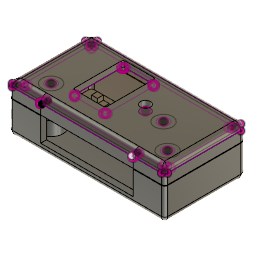
Diag_CP v4 (Autodesk Fusion 360 design; units mm, degrees)
Autodesk Fusion 360 part; units mm, degrees
sketch "Skizze1" plane through (0, 0, 0) normal (0, 0, 1) x (1, 0, 0)
  line L0 (14.5161, 23.538) -> (14.5161, 23.6029)
  line L1 (14.5161, 23.6029) -> (14.581, 23.6029)
  arc A0 (15.5262, 23.0188) -> (15.3315, 23.2135) centre (15.3315, 23.0188) ccw
  line L2 (16.0356, 22.6293) -> (16.0356, 23.0188)
  arc A1 (16.0356, 22.6293) -> (16.2303, 22.4346) centre (16.2303, 22.6293) ccw
  line L3 (16.2303, 23.2135) -> (16.5549, 23.2135)
  line L4 (13.7104, 22.4346) -> (13.3858, 22.4346)
  arc A2 (0, 1) -> (1, 0) centre (1, 1) ccw
  line L5 (14.0349, 23.2784) -> (14.0349, 22.7591)
  arc A3 (14.035, 23.2784) -> (13.7104, 23.603) centre (13.7104, 23.2784) ccw
  line L6 (15.3315, 23.2135) -> (15.0718, 23.2135)
  arc A4 (16.2303, 23.2135) -> (16.0356, 23.0188) centre (16.2303, 23.0188) ccw
  line L7 (16.3602, 22.0451) -> (16.1005, 22.0451)
  arc A5 (1, 25) -> (0, 24) centre (1, 24) ccw
  line L8 (15.2341, 22.4346) -> (15.5262, 22.4346)
  line L9 (30, 24) -> (30, 1)
  arc A6 (15.2341, 22.8889) -> (15.2341, 22.4345) centre (15.2341, 22.6617) ccw
  arc A7 (16.3602, 22.0451) -> (16.5549, 22.2398) centre (16.3602, 22.2398) ccw
  line L10 (16.5549, 22.4346) -> (16.2303, 22.4346)
  line L11 (14.5486, 22.4346) -> (14.5486, 23.2135)
  arc A8 (30, 24) -> (29, 25) centre (29, 24) ccw
  line L12 (14.581, 23.6029) -> (14.581, 23.538)
  line L13 (16.5549, 23.2135) -> (16.5549, 22.2398)
  line L14 (29, 0) -> (1, 0)
  line L15 (13.3858, 23.6029) -> (13.7104, 23.6029)
  line L16 (17.6911, 22.4346) -> (18.0806, 22.4346)
  line L17 (13.3858, 22.4346) -> (13.3858, 23.6029)
  line L18 (14.581, 23.538) -> (14.5161, 23.538)
  arc A9 (29, 0) -> (30, 1) centre (29, 1) ccw
  line L19 (0, 1) -> (0, 24)
  line L20 (15.5262, 22.8889) -> (15.2341, 22.8889)
  arc A10 (13.7104, 22.4345) -> (14.035, 22.7591) centre (13.7104, 22.7591) ccw
  line L21 (15.5262, 22.4346) -> (15.5262, 23.0188)
  arc A11 (18.3402, 22.824) -> (18.0806, 23.0836) centre (18.0806, 22.824) ccw
  arc A12 (22.8148, 23.0837) -> (22.9122, 23.3109) centre (22.5984, 23.3109) ccw
  arc A13 (18.834, 22.7591) -> (19.4832, 22.7591) centre (19.1586, 22.7591) ccw
  arc A14 (23.406, 23.0188) -> (23.5034, 22.5969) centre (24.3689, 23.0188) ccw
  line L22 (19.9771, 23.0837) -> (20.3665, 23.0837)
  line L23 (22.2631, 22.4346) -> (22.9122, 22.4346)
  arc A15 (19.4832, 22.7591) -> (18.834, 22.7591) centre (19.1586, 22.7591) ccw
  arc A16 (23.5034, 22.5968) -> (23.7306, 22.4345) centre (23.7306, 22.6747) ccw
  line L24 (1, 25) -> (29, 25)
  arc A17 (21.7692, 23.3109) -> (21.4771, 23.603) centre (21.4771, 23.3109) ccw
  arc A18 (21.4771, 23.603) -> (21.1201, 23.3433) centre (21.4771, 23.2277) ccw
  arc A19 (20.6261, 22.824) -> (20.3665, 23.0836) centre (20.3665, 22.824) ccw
  arc A20 (15.716, 20.6883) -> (15.7809, 21.0129) centre (15.7184, 20.8566) ccw
  line L25 (13.3858, 20.9479) -> (13.3858, 21.5971)
  arc A21 (19.4182, 23.3433) -> (18.899, 23.3433) centre (19.1586, 23.3433) ccw
  line L26 (22.8148, 23.0837) -> (22.2631, 22.4346)
  line L27 (18.3402, 22.6942) -> (18.3402, 22.824)
  line L28 (17.6911, 23.0837) -> (17.6911, 23.6029)
  arc A22 (13.6454, 21.8567) -> (13.3858, 21.5971) centre (13.6454, 21.5971) ccw
  arc A23 (14.5516, 21.1427) -> (14.5516, 20.6883) centre (14.5516, 20.9155) ccw
  arc A24 (17.3403, 20.883) -> (17.535, 20.6883) centre (17.535, 20.883) ccw
  line L29 (17.3402, 20.883) -> (17.3402, 21.2076)
  arc A25 (22.9122, 23.3109) -> (22.6201, 23.603) centre (22.6201, 23.3109) ccw
  line L30 (18.0806, 23.0837) -> (17.6911, 23.0837)
  arc A26 (18.899, 23.3433) -> (19.4182, 23.3433) centre (19.1586, 23.3433) ccw
  line L31 (17.8595, 20.6883) -> (17.535, 20.6883)
  arc A27 (17.8595, 21.2076) -> (17.3403, 21.2076) centre (17.5999, 21.2076) ccw
  arc A28 (23.9578, 23.4407) -> (23.7306, 23.603) centre (23.7306, 23.3628) ccw
  arc A29 (20.4964, 23.603) -> (19.9771, 23.0837) centre (20.4964, 23.0837) ccw
  line L32 (14.5516, 20.6883) -> (14.8437, 20.6883)
  line L33 (21.1201, 22.4346) -> (21.7692, 22.4346)
  line L34 (21.6718, 23.0837) -> (21.1201, 22.4346)
  line L35 (20.6262, 22.824) -> (20.6262, 22.7591)
  line L36 (13.6454, 21.8567) -> (13.9051, 21.8567)
  arc A30 (23.5035, 23.4407) -> (23.4061, 23.0188) centre (24.3689, 23.0188) ccw
  line L37 (17.6911, 23.6029) -> (18.3402, 23.6029)
  line L38 (15.7809, 21.0129) -> (15.4564, 21.1427)
  line L39 (14.8437, 20.6883) -> (14.8437, 21.2725)
  arc A31 (19.977, 22.7591) -> (20.6262, 22.7591) centre (20.3016, 22.7591) ccw
  line L40 (19.9771, 22.7591) -> (19.9771, 23.0837)
  arc A32 (22.6201, 23.603) -> (22.2631, 23.3433) centre (22.6201, 23.2277) ccw
  arc A33 (24.0552, 23.0188) -> (23.9578, 23.4407) centre (23.0923, 23.0188) ccw
  arc A34 (18.0806, 22.4346) -> (18.3402, 22.6942) centre (18.0806, 22.6942) ccw
  arc A35 (23.7306, 23.603) -> (23.5034, 23.4407) centre (23.7306, 23.3628) ccw
  arc A36 (21.6718, 23.0837) -> (21.7692, 23.3109) centre (21.4554, 23.3109) ccw
  arc A37 (19.7787, 20.883) -> (19.9734, 20.6883) centre (19.9734, 20.883) ccw
  line L41 (13.3858, 19.1008) -> (13.3858, 20.2692)
  line L42 (18.958, 21.4672) -> (19.3475, 21.4672)
  line L43 (16.3756, 19.1008) -> (16.3756, 19.1657)
  line L44 (13.7104, 19.6201) -> (13.3858, 19.6201)
  line L45 (20.2979, 21.2076) -> (20.2979, 21.0778)
  line L46 (15.7223, 19.1008) -> (15.9819, 19.8797)
  arc A38 (13.7104, 19.62) -> (13.7104, 20.2692) centre (13.7104, 19.9446) ccw
  line L47 (18.5587, 20.6883) -> (18.6236, 20.6883)
  arc A39 (18.364, 20.883) -> (18.5587, 20.6883) centre (18.5587, 20.883) ccw
  line L48 (14.5101, 19.2955) -> (14.5101, 19.6201)
  line L49 (15.0294, 19.6201) -> (15.0294, 19.4903)
  line L50 (15.0294, 19.1008) -> (14.7049, 19.1008)
  arc A40 (16.7066, 20.6883) -> (16.7715, 21.0129) centre (16.709, 20.8566) ccw
  line L51 (19.2826, 20.6883) -> (19.3475, 20.6883)
  arc A41 (18.045, 20.1069) -> (17.8178, 20.2692) centre (17.8178, 20.029) ccw
  arc A42 (20.2979, 21.2076) -> (19.7787, 21.2076) centre (20.0383, 21.2076) ccw
  arc A43 (23.7306, 22.4345) -> (23.9578, 22.5968) centre (23.7306, 22.6747) ccw
  arc A44 (16.804, 21.4023) -> (16.5119, 21.4672) centre (16.5014, 20.7302) ccw
  line L52 (17.8595, 21.2076) -> (17.8595, 21.0778)
  arc A45 (16.5119, 21.4672) -> (16.447, 21.1426) centre (16.5095, 21.2989) ccw
  line L53 (20.2979, 21.0778) -> (19.7786, 21.0778)
  line L54 (16.4405, 19.1657) -> (16.4405, 19.1008)
  arc A46 (19.0879, 20.883) -> (19.2826, 20.6883) centre (19.2826, 20.883) ccw
  arc A47 (14.5102, 19.2955) -> (14.7049, 19.1008) centre (14.7049, 19.2955) ccw
  line L55 (16.3756, 19.1657) -> (16.4405, 19.1657)
  line L56 (13.9051, 20.6883) -> (13.6454, 20.6883)
  arc A48 (15.3591, 20.7532) -> (15.7161, 20.6883) centre (15.7318, 21.789) ccw
  line L57 (18.2341, 21.4672) -> (18.6236, 21.4672)
  line L58 (14.0349, 19.1008) -> (13.7753, 19.6201)
  line L59 (14.649, 21.4672) -> (14.3894, 21.4672)
  arc A49 (15.8134, 21.4023) -> (15.5213, 21.4672) centre (15.5108, 20.7302) ccw
  arc A50 (14.8437, 21.2725) -> (14.649, 21.4672) centre (14.649, 21.2725) ccw
  arc A51 (16.3497, 20.7532) -> (16.7067, 20.6883) centre (16.7224, 21.789) ccw
  arc A52 (13.3858, 20.9479) -> (13.6454, 20.6883) centre (13.6454, 20.9479) ccw
  line L60 (18.3639, 21.8567) -> (18.3639, 20.883)
  line L61 (17.8595, 21.0778) -> (17.3402, 21.0778)
  arc A53 (23.9578, 22.5969) -> (24.0552, 23.0188) centre (23.0923, 23.0188) ccw
  arc A54 (15.5213, 21.4672) -> (15.4564, 21.1426) centre (15.5189, 21.2989) ccw
  line L62 (16.7715, 21.0129) -> (16.447, 21.1427)
  line L63 (14.8437, 21.1427) -> (14.5516, 21.1427)
  line L64 (23.471, 22.6942) -> (23.9903, 23.3433)
  arc A55 (3.2018, 4.9043) -> (2.8406, 5.2655) centre (2.8406, 4.9043) ccw
  arc A56 (15.0294, 19.6201) -> (14.5102, 19.6201) centre (14.7698, 19.6201) ccw
  line L65 (20.8245, 18.0396) -> (20.8245, 17.5204)
  arc A57 (18.1424, 19.685) -> (18.045, 20.1069) centre (17.1795, 19.685) ccw
  line L66 (2.2987, 4.814) -> (2.2987, 5.2656)
  line L67 (2.2987, 5.2656) -> (2.8406, 5.2656)
  arc A58 (17.4932, 19.685) -> (17.5906, 19.2631) centre (18.4561, 19.685) ccw
  arc A59 (17.8178, 19.1008) -> (18.045, 19.2631) centre (17.8178, 19.341) ccw
  arc A60 (21.6884, 17.715) -> (21.6884, 18.3642) centre (21.6884, 18.0396) ccw
  line L68 (3.2018, 4.9043) -> (3.2018, 4.814)
  line L69 (19.0878, 21.8567) -> (19.0878, 20.883)
  line L70 (15.4626, 19.8797) -> (15.7223, 19.1008)
  line L71 (21.3638, 18.3642) -> (21.6884, 18.3642)
  line L72 (18.6909, 18.0396) -> (18.6909, 17.5204)
  line L73 (16.7196, 17.1958) -> (16.7196, 18.3642)
  line L74 (21.91, 0.1) -> (21.91, -1)
  line L75 (19.18, -1) -> (19.18, 0)
  arc A61 (17.5907, 20.1069) -> (17.4933, 19.685) centre (18.4561, 19.685) ccw
  line L76 (16.7196, 18.3642) -> (17.109, 17.7151)
  line L77 (17.109, 17.7151) -> (17.4985, 18.3642)
  arc A62 (2.2987, 4.814) -> (3.2019, 4.814) centre (2.7503, 4.814) ccw
  line L78 (19.7786, 20.883) -> (19.7786, 21.2076)
  line L79 (18.0418, 17.5204) -> (18.0418, 18.0396)
  line L80 (15.0294, 19.4903) -> (14.5101, 19.4903)
  line L81 (17.4985, 18.3642) -> (17.4985, 17.1958)
  arc A63 (20.8245, 18.0396) -> (20.1753, 18.0396) centre (20.4999, 18.0396) ccw
  line L82 (26.905, 5.6268) -> (27.3565, 5.9881)
  line L83 (27.3565, 5.9881) -> (27.3565, 4.3624)
  line L84 (19.1086, 18.3642) -> (19.7577, 18.3642)
  arc A64 (17.5906, 19.2631) -> (17.8178, 19.1008) centre (17.8178, 19.341) ccw
  line L85 (17.5581, 19.3604) -> (18.0774, 20.0096)
  arc A65 (18.6909, 18.0396) -> (18.0417, 18.0396) centre (18.3663, 18.0396) ccw
  arc A66 (17.8178, 20.2692) -> (17.5906, 20.1069) centre (17.8178, 20.029) ccw
  arc A67 (18.0417, 17.5204) -> (18.6909, 17.5204) centre (18.3663, 17.5204) ccw
  arc A68 (20.1753, 17.5204) -> (20.8245, 17.5204) centre (20.4999, 17.5204) ccw
  line L86 (16.4405, 19.1008) -> (16.3756, 19.1008)
  line L87 (13.3858, 20.2692) -> (13.7104, 20.2692)
  line L88 (20.2979, 20.6883) -> (19.9734, 20.6883)
  line L89 (19.4331, 17.1958) -> (19.4331, 18.3642)
  arc A69 (3.0212, 5.9881) -> (2.2987, 5.2656) centre (3.0212, 5.2656) ccw
  line L90 (21.3638, 17.1958) -> (21.3638, 18.3642)
  line L91 (26.905, 4.3624) -> (27.8081, 4.3624)
  arc A70 (18.045, 19.2631) -> (18.1424, 19.685) centre (17.1795, 19.685) ccw
  line L92 (20.1754, 17.5204) -> (20.1754, 18.0396)
  line L93 (19.18, 0) -> (18.68, 0)
  arc A71 (21.91, 4) -> (19.91, 4) centre (20.91, 4) ccw
  line L94 (22.64, 0) -> (22.64, -1)
  line L95 (23.87, 0.1) -> (23.87, -1)
  arc A72 (25.87, 4) -> (23.87, 4) centre (24.87, 4) ccw
  line L96 (21.6884, 17.7151) -> (21.3638, 17.7151)
  line L97 (19.91, 0.1) -> (19.91, 4)
  line L98 (25.87, 0.1) -> (25.87, -1)
  line L99 (8.53, 3) -> (8.53, 2)
  line L100 (11.26, -1) -> (11.26, 0)
  line L101 (21.91, 0.1) -> (21.91, 4)
  circle A73 centre (25.4, 15.24) radius 1.7463
  line L102 (12.49, 3) -> (12.49, 2)
  line L103 (17.95, 0.1) -> (17.95, -1)
  line L104 (13.99, 0.1) -> (13.99, -1)
  line L105 (25.87, 0.1) -> (25.87, 4)
  arc A74 (8.53, 2) -> (9.53, 2) centre (9.03, 2) ccw
  line L106 (26.6, 0) -> (26.6, -1)
  line L107 (24.37, 3) -> (24.37, 2)
  line L108 (20.41, 3) -> (20.41, 2)
  line L109 (10.03, 0.1) -> (10.03, 4)
  line L110 (15.95, 0.1) -> (15.95, -1)
  line L111 (14.72, 0) -> (14.72, -1)
  line L112 (8.03, 0.1) -> (8.03, 4)
  arc A75 (24.37, 2) -> (25.37, 2) centre (24.87, 2) ccw
  line L113 (13.99, 0.1) -> (13.99, 4)
  arc A76 (25.37, 3) -> (24.37, 3) centre (24.87, 3) ccw
  arc A77 (21.41, 3) -> (20.41, 3) centre (20.91, 3) ccw
  line L114 (27.1, 0) -> (26.6, 0)
  line L115 (25.37, 3) -> (25.37, 2)
  line L116 (21.41, 3) -> (21.41, 2)
  line L117 (19.91, 0.1) -> (19.91, -1)
  line L118 (23.87, 0.1) -> (23.87, 4)
  line L119 (22.0129, 17.1958) -> (21.7533, 17.7151)
  line L120 (23.14, -1) -> (23.14, 0)
  circle A78 centre (25.4, 15.24) radius 3.1789
  line L121 (13.49, 3) -> (13.49, 2)
  line L122 (9.53, 3) -> (9.53, 2)
  arc A79 (20.41, 2) -> (21.41, 2) centre (20.91, 2) ccw
  line L123 (27.1, -1) -> (27.1, 0)
  line L124 (23.14, 0) -> (22.64, 0)
  line L125 (7.3, 0) -> (6.8, 0)
  line L126 (4.07, 0.1) -> (4.07, 4)
  arc A80 (4.57, 2) -> (5.57, 2) centre (5.07, 2) ccw
  line L127 (16.45, 3) -> (16.45, 2)
  line L128 (17.45, 3) -> (17.45, 2)
  arc A81 (10.03, 4) -> (8.03, 4) centre (9.03, 4) ccw
  line L129 (4.57, 3) -> (4.57, 2)
  line L130 (0.05, -1) -> (0.05, 0)
  arc A82 (17.45, 3) -> (16.45, 3) centre (16.95, 3) ccw
  line L131 (17.95, 0.1) -> (17.95, 4)
  line L132 (11.99, 0.1) -> (11.99, -1)
  line L133 (7.3, -1) -> (7.3, 0)
  arc A83 (12.49, 2) -> (13.49, 2) centre (12.99, 2) ccw
  line L134 (10.03, 0.1) -> (10.03, -1)
  line L135 (3.34, 0) -> (2.84, 0)
  line L136 (15.95, 0.1) -> (15.95, 4)
  line L137 (10.76, 0) -> (10.76, -1)
  line L138 (6.07, 0.1) -> (6.07, -1)
  line L139 (-7.4, 0) -> (-7.4, -6.8)
  arc A84 (16.45, 2) -> (17.45, 2) centre (16.95, 2) ccw
  line L140 (5.57, 3) -> (5.57, 2)
  line L141 (15.22, 0) -> (14.72, 0)
  line L142 (4.07, 0.1) -> (4.07, -1)
  line L143 (37.34, 0) -> (37.34, -6.8)
  arc A85 (17.95, 4) -> (15.95, 4) centre (16.95, 4) ccw
  line L144 (11.99, 0.1) -> (11.99, 4)
  arc A86 (5.57, 3) -> (4.57, 3) centre (5.07, 3) ccw
  arc A87 (6.07, 4) -> (4.07, 4) centre (5.07, 4) ccw
  line L145 (32.39, 0) -> (29.89, 0)
  line L146 (29.89, -1) -> (0.05, -1)
  line L147 (-2.45, 0) -> (-4.15, 0)
  line L148 (-0.65, -11.6) -> (-0.65, -6.8)
  line L149 (6.8, 0) -> (6.8, -1)
  arc A88 (9.53, 3) -> (8.53, 3) centre (9.03, 3) ccw
  line L150 (11.26, 0) -> (10.76, 0)
  arc A89 (13.99, 4) -> (11.99, 4) centre (12.99, 4) ccw
  line L151 (15.22, -1) -> (15.22, 0)
  line L152 (2.84, 0) -> (2.84, -1)
  line L153 (18.68, 0) -> (18.68, -1)
  arc A90 (13.49, 3) -> (12.49, 3) centre (12.99, 3) ccw
  line L154 (0.05, 0) -> (-2.45, 0)
  line L155 (-4.15, 0) -> (-4.15, -2.8667)
  line L156 (32.39, -1.6) -> (32.39, 0)
  line L157 (34.09, -3.6853) -> (34.09, -3.548)
  line L158 (-4.15, -3.548) -> (-4.15, -3.6853)
  line L159 (-5.85, -4.2) -> (-5.85, -2.6)
  line L160 (-2.45, -1.6) -> (-2.45, 0)
  line L161 (-4.15, -4.3667) -> (-4.15, -7.2333)
  arc A91 (27.6031, 0.7808) -> (27.8627, 1.0404) centre (27.6031, 1.0404) ccw
  line L162 (-4.15, 0) -> (-5.85, 0)
  line L163 (35.79, 0) -> (34.09, 0)
  line L164 (32.39, -6.8) -> (32.39, -5.2)
  line L165 (-2.45, -4.2) -> (-2.45, -2.6)
  line L166 (27.6031, 0.7808) -> (27.4733, 0.7808)
  line L167 (34.09, -7.2333) -> (34.09, -4.3667)
  line L168 (35.79, -1.6) -> (35.79, 0)
  line L169 (37.34, 0) -> (35.79, 0)
  line L170 (34.09, 0) -> (32.39, 0)
  line L171 (35.79, -6.8) -> (35.79, -5.2)
  line L172 (-2.45, -6.8) -> (-2.45, -5.2)
  line L173 (37.34, -6.8) -> (35.79, -6.8)
  line L174 (32.39, -6.8) -> (30.59, -6.8)
  line L175 (34.09, -2.8667) -> (34.09, 0)
  line L176 (-4.15, -7.9147) -> (-4.15, -8.052)
  line L177 (3.5362, 8.38) -> (3.5362, 23.62)
  line L178 (8.03, 0.1) -> (8.03, -1)
  line L179 (3.34, -1) -> (3.34, 0)
  line L180 (6.07, 0.1) -> (6.07, 4)
  line L181 (27.8628, 1.9492) -> (27.8628, 1.0404)
  line L182 (35.79, -4.2) -> (35.79, -2.6)
  line L183 (34.09, -11.6) -> (34.09, -8.7333)
  line L184 (35.79, -6.8) -> (32.39, -6.8)
  line L185 (32.39, -4.2) -> (32.39, -2.6)
  line L186 (34.09, -8.052) -> (34.09, -7.9147)
  line L187 (-0.65, -6.8) -> (-2.45, -6.8)
  line L188 (30.59, -6.8) -> (30.59, -11.6)
  line L189 (29.89, 0) -> (29.89, -1)
  line L190 (-5.85, -6.8) -> (-7.4, -6.8)
  line L191 (30.59, -11.6) -> (-0.65, -11.6)
  line L192 (-5.85, -1.6) -> (-5.85, 0)
  line L193 (-4.15, -8.7333) -> (-4.15, -11.6)
  line L194 (-5.85, -6.8) -> (-5.85, -5.2)
  line L195 (-5.85, 0) -> (-7.4, 0)
  line L196 (-2.45, -6.8) -> (-5.85, -6.8)
  line L197 (4.965, 22.8263) -> (4.33, 22.8263)
  line L198 (11.95, 14.73) -> (12.7438, 14.73)
  line L199 (4.965, 9.65) -> (4.965, 9.1737)
  line L200 (11.4738, 14.73) -> (11.4738, 9.65)
  line L201 (6.3937, 23.62) -> (12.7438, 23.62)
  line L202 (11.4738, 17.27) -> (11.95, 17.27)
  line L203 (4.965, 9.1737) -> (4.965, 8.38)
  line L204 (4.8062, 22.35) -> (4.965, 22.35)
  line L205 (28.3901, 0.7808) -> (29.0392, 0.7808)
  line L206 (4.965, 23.62) -> (6.3937, 23.62)
  line L207 (11.4738, 22.35) -> (11.4738, 17.27)
  line L208 (6.3937, 9.65) -> (4.965, 9.65)
  line L209 (12.7438, 8.38) -> (6.3937, 8.38)
  line L210 (11.95, 17.27) -> (12.7438, 17.27)
  line L211 (11.1562, 13.1425) -> (11.1562, 13.3012)
  line L212 (11.4738, 9.65) -> (6.3937, 9.65)
  line L213 (6.3937, 22.35) -> (11.4738, 22.35)
  line L214 (11.1562, 13.3012) -> (11.1562, 13.6187)
  line L215 (11.1562, 13.7775) -> (10.8387, 13.46)
  line L216 (11.4738, 22.35) -> (11.95, 22.8263)
  line L217 (12.7438, 14.73) -> (12.7438, 8.38)
  line L218 (4.8062, 9.65) -> (4.8062, 22.35)
  line L219 (4.965, 22.8263) -> (4.965, 23.62)
  line L220 (4.965, 8.38) -> (3.5362, 8.38)
  line L221 (4.965, 9.65) -> (4.8062, 9.65)
  line L222 (3.5362, 23.62) -> (4.965, 23.62)
  line L223 (10.8387, 13.46) -> (11.1562, 13.1425)
  line L224 (28.3901, 1.6896) -> (28.7146, 1.9492)
  line L225 (6.3937, 9.1737) -> (11.95, 9.1737)
  line L226 (10.5212, 13.46) -> (11.1562, 12.825)
  arc A92 (3.5362, 22.35) -> (3.5362, 21.08) centre (3.5362, 21.715) ccw
  line L227 (11.4738, 17.27) -> (11.4738, 14.73)
  line L228 (28.7146, 1.9492) -> (28.7146, 0.7808)
  line L229 (4.965, 22.35) -> (6.3937, 22.35)
  line L230 (12.7438, 23.62) -> (12.7438, 17.27)
  line L231 (11.1562, 13.6187) -> (10.9975, 13.46)
  arc A93 (3.5362, 16.4763) -> (3.5362, 15.3651) centre (3.5362, 15.9207) ccw
  line L232 (12.7438, 17.27) -> (12.7438, 14.73)
  line L233 (6.3937, 22.35) -> (6.3937, 22.8263)
  line L234 (4.965, 22.35) -> (4.965, 22.8263)
  line L235 (6.3937, 9.1737) -> (6.3937, 8.38)
  line L236 (11.1562, 12.825) -> (11.1562, 12.9837)
  line L237 (11.4738, 14.73) -> (11.95, 14.73)
  line L238 (6.3937, 8.38) -> (4.965, 8.38)
  arc A94 (14.3179, 8.5894) -> (14.0583, 8.849) centre (14.0583, 8.5894) ccw
  arc A95 (3.5362, 10.92) -> (3.5362, 9.65) centre (3.5362, 10.285) ccw
  line L239 (4.33, 9.1737) -> (4.965, 9.1737)
  line L240 (11.95, 14.73) -> (11.95, 9.1737)
  line L241 (4.8062, 22.35) -> (4.33, 22.8263)
  line L242 (11.1562, 13.9362) -> (10.68, 13.46)
  line L243 (6.3937, 22.8263) -> (11.95, 22.8263)
  line L244 (6.3937, 9.65) -> (6.3937, 9.1737)
  line L245 (13.6688, 9.9281) -> (14.318, 9.3764)
  arc A96 (13.6689, 9.9281) -> (13.4417, 10.0255) centre (13.4417, 9.7118) ccw
  line L246 (7.124, 13.714) -> (6.616, 13.714)
  line L247 (20.955, 16.3513) -> (20.955, 16.6687)
  line L248 (7.124, 16.254) -> (6.616, 16.254)
  arc A97 (13.1495, 9.7334) -> (13.4092, 9.3764) centre (13.5248, 9.7334) ccw
  line L249 (11.1562, 13.7775) -> (11.1562, 13.9362)
  line L250 (11.1562, 13.6187) -> (11.1562, 13.7775)
  line L251 (11.95, 9.1737) -> (11.4738, 9.65)
  line L252 (11.1562, 14.095) -> (10.5212, 13.46)
  line L253 (20.8675, 16.04) -> (20.8675, 14.44)
  line L254 (9.156, 13.206) -> (9.664, 13.206)
  line L255 (6.616, 18.286) -> (7.124, 18.286)
  line L256 (10.9975, 13.46) -> (11.1562, 13.3012)
  line L257 (11.1562, 12.9837) -> (11.1562, 13.1425)
  line L258 (10.68, 13.46) -> (11.1562, 12.9837)
  line L259 (14.318, 9.3764) -> (14.318, 10.0255)
  line L260 (6.616, 13.714) -> (6.616, 13.206)
  arc A98 (20.8675, 16.04) -> (17.8675, 16.04) centre (19.3675, 15.24) ccw
  arc A99 (17.8675, 14.44) -> (20.8675, 14.44) centre (19.3675, 15.24) ccw
  line L261 (11.95, 17.27) -> (11.95, 22.8263)
  line L262 (6.3937, 22.8263) -> (6.3937, 23.62)
  line L263 (14.318, 8.5894) -> (14.318, 8.4596)
  line L264 (9.156, 18.286) -> (9.664, 18.286)
  line L265 (6.616, 15.746) -> (7.124, 15.746)
  line L266 (7.124, 15.746) -> (7.124, 16.254)
  line L267 (4.33, 9.1737) -> (4.8062, 9.65)
  line L268 (9.664, 13.206) -> (9.664, 13.714)
  line L269 (4.33, 9.1737) -> (4.33, 22.8263)
  line L270 (6.616, 16.254) -> (6.616, 15.746)
  line L271 (9.664, 15.746) -> (9.664, 16.254)
  line L272 (11.1562, 13.9362) -> (11.1562, 14.095)
  line L273 (7.124, 18.794) -> (6.616, 18.794)
  line L274 (17.3687, 9.4241) -> (17.3687, 9.0996)
  arc A100 (17.3687, 9.4241) -> (16.7195, 9.4241) centre (17.0441, 9.4241) ccw
  line L275 (9.664, 13.714) -> (9.156, 13.714)
  line L276 (9.664, 18.794) -> (9.156, 18.794)
  line L277 (9.156, 13.714) -> (9.156, 13.206)
  line L278 (20.0056, 15.0869) -> (20.0056, 15.6091)
  arc A101 (20.2144, 15.8179) -> (20.0056, 15.6091) centre (20.2144, 15.6091) ccw
  line L279 (18.0056, 14.8781) -> (18.3189, 15.8179)
  line L280 (9.664, 16.254) -> (9.156, 16.254)
  line L281 (16.3513, 15.7264) -> (16.0973, 16.0439)
  line L282 (7.124, 13.206) -> (7.124, 13.714)
  line L283 (9.156, 16.254) -> (9.156, 15.746)
  arc A102 (13.4417, 10.0255) -> (13.1496, 9.7334) centre (13.4417, 9.7334) ccw
  line L284 (7.124, 18.286) -> (7.124, 18.794)
  line L285 (17.7213, 16.3513) -> (17.7213, 16.6687)
  line L286 (16.4148, 15.1803) -> (16.9228, 15.1803)
  line L287 (6.616, 18.794) -> (6.616, 18.286)
  line L288 (9.156, 18.794) -> (9.156, 18.286)
  line L289 (9.664, 18.286) -> (9.664, 18.794)
  arc A103 (17.2403, 14.8628) -> (16.9228, 15.1803) centre (16.9228, 14.8628) ccw
  line L290 (16.0973, 14.5453) -> (16.0973, 14.8628)
  line L291 (18.5538, 15.1131) -> (18.0839, 15.1131)
  arc A104 (17.8675, 16.04) -> (17.8675, 14.44) centre (19.3675, 15.24) ccw
  line L292 (9.156, 15.746) -> (9.664, 15.746)
  arc A105 (16.4148, 15.1803) -> (16.0973, 14.8628) centre (16.4148, 14.8628) ccw
  line L293 (17.2402, 15.7264) -> (17.2402, 16.3614)
  arc A106 (17.8675, 14.44) -> (20.8675, 14.44) centre (19.3675, 15.24) ccw
  line L294 (17.2402, 14.5453) -> (16.0973, 14.5453)
  line L295 (13.1496, 8.8491) -> (14.0583, 8.8491)
  line L296 (6.616, 13.206) -> (7.124, 13.206)
  line L297 (16.7196, 9.0996) -> (16.7196, 9.4241)
  line L298 (17.888, 10.2352) -> (17.888, 10.8843)
  line L299 (20.2144, 15.8179) -> (20.4233, 15.8179)
  line L300 (17.2402, 13.5572) -> (17.2402, 14.0653)
  line L301 (18.3189, 15.8179) -> (18.6321, 14.8781)
  circle A107 centre (19.3675, 10.0013) radius 1.27
  line L302 (17.2402, 14.8628) -> (17.2402, 14.5453)
  line L303 (17.888, 9.7487) -> (17.3687, 9.489)
  arc A108 (20.8675, 16.04) -> (17.8675, 16.04) centre (19.3675, 15.24) ccw
  line L304 (17.888, 9.0996) -> (16.7196, 9.0996)
  arc A109 (20.0056, 15.0869) -> (20.2144, 14.8781) centre (20.2144, 15.0869) ccw
  line L305 (17.88, 16.51) -> (17.5625, 16.51)
  line L306 (19.3675, 10.795) -> (19.3675, 11.7157)
  line L307 (16.7196, 10.5597) -> (17.888, 10.5597)
  line L308 (16.0973, 16.0439) -> (17.2402, 16.0439)
  line L309 (16.9792, 10.2352) -> (16.7196, 10.5597)
  circle A110 centre (19.3675, 15.24) radius 1.5
  line L310 (20.4233, 14.8781) -> (20.2144, 14.8781)
  line L311 (16.0973, 13.5572) -> (17.2402, 13.5572)
  dimension "d1" = 30
  dimension "d2" = 25
  measures "d1" distance of A5.end L9.start
  measures "d2" distance of A8.end L14.start
ref_plane "Arbeitsebene1" through (15, 12.5, -3) normal (0, 0, 1) x (1, 0, 0)
sketch "Skizze2" plane through (15, 12.5, -3) normal (0, 0, 1) x (1, 0, 0)
  line L0 (-14, 12.5) -> (14, 12.5)
  arc A0 (-14, 12.5) -> (-15, 11.5) centre (-14, 11.5) ccw
  line L1 (-15, -11.5) -> (-15, 11.5)
  arc A1 (15, 11.5) -> (14, 12.5) centre (14, 11.5) ccw
  line L2 (15, 11.5) -> (15, -11.5)
  arc A2 (14, -12.5) -> (15, -11.5) centre (14, -11.5) ccw
  line L3 (14, -12.5) -> (-14, -12.5)
  arc A3 (-15, -11.5) -> (-14, -12.5) centre (-14, -11.5) ccw
  circle A4 centre (4.3675, 2.74) radius 1.5
  circle A5 centre (10.4, 2.74) radius 1.7463
  line L4 (-11.4638, 11.12) -> (-10.035, 11.12)
  line L5 (-10.035, 11.12) -> (-8.6063, 11.12)
  line L6 (-8.6063, 11.12) -> (-2.2562, 11.12)
  line L7 (-2.2562, 11.12) -> (-2.2562, 4.77)
  line L8 (-2.2562, 4.77) -> (-2.2562, 2.23)
  line L9 (-2.2562, 2.23) -> (-2.2562, -4.12)
  line L10 (-2.2562, -4.12) -> (-8.6063, -4.12)
  line L11 (-8.6063, -4.12) -> (-10.035, -4.12)
  line L12 (-10.035, -4.12) -> (-11.4638, -4.12)
  line L13 (-11.4638, -4.12) -> (-11.4638, 11.12)
  line L14 (-25, -12.5) -> (25, -12.5)
  line L15 (26, -11.5) -> (26, 13)
  line L16 (24, 15) -> (-24, 15)
  line L17 (-26, 13) -> (-26, -11.5)
  circle A6 centre (10.4, 2.74) radius 4
  circle A7 centre (10.4, 2.74) radius 1.75
  line L18 (-11.7638, 11.92) -> (-1.9562, 11.92)
  line L19 (-1.4562, 11.42) -> (-1.4562, -4.42)
  line L20 (-1.9562, -4.92) -> (-11.7638, -4.92)
  line L21 (-12.2638, -4.42) -> (-12.2638, 11.42)
  arc A8 (-12.2638, -4.42) -> (-11.7638, -4.92) centre (-11.7638, -4.42) ccw
  arc A9 (-1.9562, -4.92) -> (-1.4562, -4.42) centre (-1.9562, -4.42) ccw
  arc A10 (-1.4562, 11.42) -> (-1.9562, 11.92) centre (-1.9562, 11.42) ccw
  arc A11 (-11.7638, 11.92) -> (-12.2638, 11.42) centre (-11.7638, 11.42) ccw
  circle A12 centre (4.3675, 2.74) radius 1.65
  arc A13 (-24, 15) -> (-26, 13) centre (-24, 13) ccw
  arc A14 (26, 13) -> (24, 15) centre (24, 13) ccw
  arc A15 (25, -12.5) -> (26, -11.5) centre (25, -11.5) ccw
  arc A16 (-26, -11.5) -> (-25, -12.5) centre (-25, -11.5) ccw
  line L22 (-15.5, 8.5) -> (-13.5, 8.5)
  line L23 (-13.5, 8.5) -> (-13.5, 6.5)
  line L24 (-13.5, 6.5) -> (-15.5, 6.5)
  line L25 (-15.5, 6.5) -> (-15.5, 8.5)
  line L26 (-15.5, 8.5) -> (-17.5, 8.5)
  line L27 (-17.5, 8.5) -> (-17.5, 6.5)
  line L28 (-17.5, 6.5) -> (-15.5, 6.5)
  line L29 (-15.5, 6.5) -> (-15.5, 8.5)
  circle A17 centre (-19.5, -5) radius 4
  line L30 (-24, 12) -> (-24, -9.5)
  line L31 (-23, -10.5) -> (23, -10.5)
  line L32 (24, -9.5) -> (24, 12)
  line L33 (23, 13) -> (-23, 13)
  circle A18 centre (-19.5, -5) radius 3
  circle A19 centre (-19.5, -5) radius 1.75
  circle A20 centre (19.5, -5) radius 4
  circle A21 centre (19.5, -5) radius 3
  circle A22 centre (19.5, -5) radius 1.75
  arc A23 (-23, 13) -> (-24, 12) centre (-23, 12) ccw
  arc A24 (24, 12) -> (23, 13) centre (23, 12) ccw
  arc A25 (23, -10.5) -> (24, -9.5) centre (23, -9.5) ccw
  arc A26 (-24, -9.5) -> (-23, -10.5) centre (-23, -9.5) ccw
  line L34 (-15.5, -10.5) -> (-15.5, -12.5)
  line L35 (15.5, -10.5) -> (15.5, -12.5)
  line L36 (-24.8, 12) -> (-24.8, -9.5)
  arc A27 (-24.8, -9.5) -> (-23, -11.3) centre (-23, -9.5) ccw
  line L37 (-23, -11.3) -> (23, -11.3)
  arc A28 (23, -11.3) -> (24.8, -9.5) centre (23, -9.5) ccw
  line L38 (24.8, -9.5) -> (24.8, 12)
  arc A29 (24.8, 12) -> (23, 13.8) centre (23, 12) ccw
  line L39 (23, 13.8) -> (-23, 13.8)
  arc A30 (-23, 13.8) -> (-24.8, 12) centre (-23, 12) ccw
  dimension "d4" = 11
  dimension "d5" = 11
  dimension "d6" = 2.5
  dimension "d7" = 8
  dimension "d8" = 3.5
  dimension "d9" = 0.8
  dimension "d10" = 0.8
  dimension "d11" = 0.8
  dimension "d12" = 0.8
  dimension "d13" = 0.5
  dimension "d14" = 0.5
  dimension "d15" = 0.5
  dimension "d16" = 0.5
  dimension "d17" = 3.3
  dimension "d18" = 2
  dimension "d19" = 2
  dimension "d20" = 1
  dimension "d21" = 1
  dimension "d22" = 2
  dimension "d23" = 0.5
  dimension "d24" = 2
  dimension "d25" = 2
  dimension "d26" = 4
  dimension "d27" = 8
  dimension "d29" = 6
  dimension "d30" = 3.5
  dimension "d31" = 8
  dimension "d32" = 6
  dimension "d33" = 3.5
  dimension "d34" = 7.5
  dimension "d35" = 6.5
  dimension "d36" = 6.5
  dimension "d37" = 7.5
  dimension "d38" = 1
  dimension "d39" = 1
  dimension "d40" = 1
  dimension "d41" = 1
  dimension "d42" = 2
  dimension "d43" = 0.5
  dimension "d44" = 0.5
  dimension "d45" = 2
  dimension "d46" = 2
  dimension "d47" = 2
  dimension "d48" = 0.8
  constraint horizontal L14
  constraint vertical L15
  constraint horizontal L16
  constraint vertical L17
  constraint concentric A5 A6
  constraint concentric A5 A7
  constraint horizontal L18
  constraint vertical L19
  constraint horizontal L20
  constraint vertical L21
  constraint tangent L20 A8
  constraint tangent L21 A8
  constraint tangent L19 A9
  constraint tangent L20 A9
  constraint tangent L18 A10
  constraint tangent L19 A10
  constraint tangent L18 A11
  constraint tangent L21 A11
  constraint concentric A4 A12
  constraint tangent L16 A13
  constraint tangent L17 A13
  constraint tangent L15 A14
  constraint tangent L16 A14
  constraint tangent L14 A15
  constraint tangent L15 A15
  constraint tangent L14 A16
  constraint tangent L17 A16
  constraint collinear L3 L14
  constraint horizontal L22
  constraint vertical L23
  constraint horizontal L24
  constraint vertical L25
  constraint horizontal L26
  constraint vertical L27
  constraint horizontal L28
  constraint vertical L29
  constraint collinear L24 L28
  constraint concentric A17 A18
  constraint concentric A17 A19
  constraint concentric A20 A21
  constraint concentric A20 A22
  constraint parallel L17 L30
  constraint parallel L14 L31
  constraint parallel L15 L32
  constraint parallel L16 L33
  constraint tangent L30 A23
  constraint tangent L33 A23
  constraint tangent L33 A24
  constraint tangent L32 A24
  constraint tangent L31 A25
  constraint tangent L32 A25
  constraint tangent L31 A26
  constraint tangent L30 A26
  constraint coincident L31 L34.start
  constraint coincident L14 L34.end
  constraint perpendicular L14 L34
  constraint coincident L31 L35.start
  constraint perpendicular L31 L35
  measures "d4" distance of L2 L15
  measures "d5" distance of L1 L17
  measures "d6" distance of L0 L16
  measures "d7" diameter of A6
  measures "d8" diameter of A7
  measures "d9" distance of L9.end L19
  measures "d10" distance of L12.end L21
  measures "d11" distance of L6.end L18
  measures "d12" distance of L9.end L20
  measures "d13" radius of A8
  measures "d14" radius of A9
  measures "d15" radius of A10
  measures "d16" radius of A11
  measures "d17" diameter of A12
  measures "d18" radius of A13
  measures "d19" radius of A14
  measures "d20" radius of A15
  measures "d21" radius of A16
  measures "d22" distance of L22.start L22.end
  measures "d23" distance of L1 L24.end
  measures "d24" distance of L22.end L23.end
  measures "d25" distance of L22.start L26.end
  measures "d26" distance of L0.start L22
  measures "d27" diameter of A17
  measures "d29" diameter of A18
  measures "d30" diameter of A19
  measures "d31" diameter of A20
  measures "d32" diameter of A21
  measures "d33" diameter of A22
  measures "d34" distance of L14 A17.centre
  measures "d35" distance of L17 A17.centre
  measures "d36" distance of L15 A20.centre
  measures "d37" distance of L14 A20.centre
  measures "d38" radius of A23
  measures "d39" radius of A24
  measures "d40" radius of A25
  measures "d41" radius of A26
  measures "d42" distance of L14 L31
  measures "d43" distance of L1 L34
  measures "d44" distance of L2 L35.start
  measures "d45" distance of L15 L32
  measures "d46" distance of L16 L33
  measures "d47" distance of L17 L30
extrude "Extrusion1" add sketch "Skizze2" against normal blind 2 contours L0 A0 L1 A1 L2 L22 L24 L26 L27 L28 L30 L31 L32 L33 A23 A24 A25 A26 | L0 A0 L1 A1 L2 L22 L23 L24 L31 | L1 L22 L23 L24 | L1 L22 L24 L25 L29 | L2 L31 L35 L37 | L1 L2 L31 L37 | L25 L26 L27 L28 L29 | L2 A2 L14 L35 L37 | L1 L2 A2 L3 A3 L14 L37 | L1 L31 L34 L37 | L30 L31 L32 L33 A23 A24 A25 A26 L34 L35 L36 A27 L37 A28 L38 A29 L39 A30 | L1 A3 L14 L34 L37 | L14 L15 L16 L17 A13 A14 A15 A16 L34 L35 L36 A27 L37 A28 L38 A29 L39 A30 | A4 | L4 L5 L6 L7 L8 L9 L10 L11 L12 L13 | A6 | L18 L19 L20 L21 A8 A9 A10 A11 | A12 | A17 | A18 | A20 | A21 makes body 1
extrude "Extrusion2" add sketch "Skizze2" along normal blind 1 contours L2 L31 L35 L37 | L1 L2 L31 L37 | L2 A2 L14 L35 L37 | L1 L2 A2 L3 A3 L14 L37 | L1 L31 L34 L37 | L1 A3 L14 L34 L37 bodies 1
extrude "Extrusion3" add sketch "Skizze2" along normal blind 9 contours L14 L15 L16 L17 A13 A14 A15 A16 L34 L35 L36 A27 L37 A28 L38 A29 L39 A30 bodies 1
extrude "Extrusion4" add sketch "Skizze2" along normal blind 10 contours L30 L31 L32 L33 A23 A24 A25 A26 L34 L35 L36 A27 L37 A28 L38 A29 L39 A30 bodies 1
extrude "Extrusion5" add sketch "Skizze2" along normal blind 3 contours A6 bodies 1
extrude "Extrusion6" add sketch "Skizze2" along normal blind 3 contours L1 L22 L23 L24 | L1 L22 L24 L25 L29 bodies 1
extrude "Extrusion7" add sketch "Skizze2" along normal blind 4.5 contours L25 L26 L27 L28 L29 bodies 1
extrude "Extrusion8" add sketch "Skizze2" along normal blind 4.6 contours A17 | A18 | A20 | A21 bodies 1
chamfer "Fase1" distance 1 angle 45 1 edges at (21.6707, 13.7935, 0) on bodies 1
sketch "Skizze3" plane through (0, 0, -5) normal (0, 0, -1) x (1, 0, 0)
  circle A0 centre (-4.5, -7.5) radius 1.75
  circle A1 centre (34.5, -7.5) radius 1.75
  circle A2 centre (25.4, -15.24) radius 1.7463
  arc A3 (-10, 0) -> (-11, -1) centre (-10, -1) ccw
  line L0 (-11, -1) -> (-11, -25.5)
  arc A4 (-11, -25.5) -> (-9, -27.5) centre (-9, -25.5) ccw
  line L1 (-9, -27.5) -> (39, -27.5)
  arc A5 (39, -27.5) -> (41, -25.5) centre (39, -25.5) ccw
  line L2 (41, -25.5) -> (41, -1)
  arc A6 (41, -1) -> (40, 0) centre (40, -1) ccw
  line L3 (40, 0) -> (-10, 0)
  circle A7 centre (-4.5, -7.5) radius 3
  circle A8 centre (25.4, -15.24) radius 3
  circle A9 centre (34.5, -7.5) radius 3
  dimension "d66" = 6
  dimension "d67" = 6
  dimension "d68" = 6
  constraint concentric A0 A7
  constraint concentric A2 A8
  constraint concentric A1 A9
  measures "d66" diameter of A7
  measures "d67" diameter of A8
  measures "d68" diameter of A9
extrude "Extrusion9" cut sketch "Skizze3" against normal blind 1.5 contours A7 | A8 | A9 bodies 1
fillet "Abrundung1" radius 1 2 edges at (-2.5, 20, -3) (-0.5, 19, -3) on bodies 1
fillet "Abrundung2" radius 1 2 edges at (-1, 21, -3) (1.5, 19.5, -3) on bodies 1
fillet "Abrundung3" radius 2 8 edges at (-11, 13.25, -5) (-10.4142, 26.9142, -5) (15, 27.5, -5) (40.4142, 26.9142, -5) (41, 13.25, -5) (40.7071, 0.2929, -5) (15, 0, -5) (-10.7071, 0.2929, -5) on bodies 1
ref_plane "Arbeitsebene2" through (15, 12.5, 9.6) normal (0, 0, 1) x (1, 0, 0)
sketch "Skizze4" plane through (15, 12.5, 9.6) normal (0, 0, 1) x (1, 0, 0)
  line L0 (-15.5, -12.5) -> (15.5, -12.5)
  line L1 (15.5, -12.5) -> (25, -12.5)
  arc A0 (25, -12.5) -> (26, -11.5) centre (25, -11.5) ccw
  line L2 (26, -11.5) -> (26, 13)
  arc A1 (26, 13) -> (24, 15) centre (24, 13) ccw
  line L3 (24, 15) -> (-24, 15)
  arc A2 (-24, 15) -> (-26, 13) centre (-24, 13) ccw
  line L4 (-26, 13) -> (-26, -11.5)
  arc A3 (-26, -11.5) -> (-25, -12.5) centre (-25, -11.5) ccw
  line L5 (-25, -12.5) -> (-15.5, -12.5)
  line L6 (15.5, -10.5) -> (-15.5, -10.5)
  line L7 (23, -10.5) -> (15.5, -10.5)
  arc A4 (23, -10.5) -> (24, -9.5) centre (23, -9.5) ccw
  line L8 (24, 12) -> (24, -9.5)
  arc A5 (24, 12) -> (23, 13) centre (23, 12) ccw
  line L9 (-23, 13) -> (23, 13)
  arc A6 (-23, 13) -> (-24, 12) centre (-23, 12) ccw
  line L10 (-24, -9.5) -> (-24, 12)
  arc A7 (-24, -9.5) -> (-23, -10.5) centre (-23, -9.5) ccw
  line L11 (-15.5, -11.3) -> (-15.5, -10.5)
  line L12 (-15.5, -10.5) -> (-23, -10.5)
  line L13 (15.5, -10.5) -> (15.5, -11.3)
  circle A8 centre (10.4, 2.74) radius 1.75
  circle A9 centre (19.5, -5) radius 1.75
  circle A10 centre (-19.5, -5) radius 1.75
  circle A11 centre (4.3675, 2.74) radius 1.5
  line L14 (-12.2638, -4.42) -> (-12.2638, 11.42)
  line L15 (-11.7638, 11.92) -> (-1.9562, 11.92)
  arc A12 (-11.7638, 11.92) -> (-12.2638, 11.42) centre (-11.7638, 11.42) ccw
  line L16 (-1.4562, 11.42) -> (-1.4562, -4.42)
  arc A13 (-1.4562, 11.42) -> (-1.9562, 11.92) centre (-1.9562, 11.42) ccw
  arc A14 (-1.9562, -4.92) -> (-1.4562, -4.42) centre (-1.9562, -4.42) ccw
  line L17 (-1.9562, -4.92) -> (-11.7638, -4.92)
  arc A15 (-12.2638, -4.42) -> (-11.7638, -4.92) centre (-11.7638, -4.42) ccw
  line L18 (-15, -10.5) -> (-15, -12.5)
  line L19 (15, -10.5) -> (15, -12.5)
  circle A16 centre (4.3675, 2.74) radius 1.65
  circle A17 centre (10.4, 2.74) radius 1.25
  circle A18 centre (10.4, 2.74) radius 3
  circle A19 centre (19.5, -5) radius 1.25
  circle A20 centre (19.5, -5) radius 3
  circle A21 centre (-19.5, -5) radius 1.25
  circle A22 centre (-19.5, -5) radius 3
  line L20 (15.5, -11.7) -> (25, -11.7)
  arc A23 (25, -11.7) -> (25.2, -11.5) centre (25, -11.5) ccw
  line L21 (25.2, -11.5) -> (25.2, 13)
  arc A24 (25.2, 13) -> (24, 14.2) centre (24, 13) ccw
  line L22 (24, 14.2) -> (-24, 14.2)
  arc A25 (-24, 14.2) -> (-25.2, 13) centre (-24, 13) ccw
  line L23 (-25.2, 13) -> (-25.2, -11.5)
  arc A26 (-25.2, -11.5) -> (-25, -11.7) centre (-25, -11.5) ccw
  line L24 (-25, -11.7) -> (-15.5, -11.7)
  line L25 (-15.5, -11.7) -> (15.5, -11.7)
  point P0 (24.8, -9.5)
  point P1 (-23, -10.5)
  point P2 (-11.7638, 11.42)
  point P3 (-1.9562, 11.42)
  dimension "d75" = 0.5
  dimension "d76" = 0.5
  dimension "d77" = 3.3
  dimension "d78" = 2.5
  dimension "d79" = 6
  dimension "d80" = 2.5
  dimension "d81" = 6
  dimension "d82" = 2.5
  dimension "d83" = 6
  dimension "d84" = -0.8
  constraint coincident L6 L18.start
  constraint coincident L0 L18.end
  constraint perpendicular L0 L18
  constraint coincident L6 L19.start
  constraint perpendicular L6 L19
  constraint concentric A11 A16
  constraint concentric A8 A17
  constraint concentric A8 A18
  constraint concentric A9 A19
  constraint concentric A9 A20
  constraint concentric A10 A21
  constraint concentric A21 A22
  measures "d75" distance of L6.end L18.start
  measures "d76" distance of L6.start L19.start
  measures "d77" diameter of A16
  measures "d78" diameter of A17
  measures "d79" diameter of A18
  measures "d80" diameter of A19
  measures "d81" diameter of A20
  measures "d82" diameter of A21
  measures "d83" diameter of A22
extrude "Extrusion10" add sketch "Skizze4" along normal blind 2 separate body contours L0 L1 A0 L2 A1 L3 A2 L4 A3 L5 L18 L19 L20 A23 L21 A24 L22 A25 L23 A26 L24 L25 | L0 L18 L19 L25 | L6 L7 A4 L8 A5 L9 A6 L10 A7 L12 L18 L19 L20 A23 L21 A24 L22 A25 L23 A26 L24 L25 | L6 L18 L19 L25 | L6 L7 A4 L8 A5 L9 A6 L10 A7 L12 | A8 | A9 | A10 | A17 | A18 | A19 | A20 | A21 | A22 makes body 2
fillet "Abrundung4" radius 2 10 edges at (-11, 13.25, 11.6) (-10.7071, 0.2929, 11.6) (-5.25, 0, 11.6) (15, 0, 11.6) (35.25, 0, 11.6) (40.7071, 0.2929, 11.6) (41, 13.25, 11.6) (40.4142, 26.9142, 11.6) (15, 27.5, 11.6) (-10.4142, 26.9142, 11.6) on bodies 2
extrude "Extrusion11" add sketch "Skizze4" against normal blind 3.4 separate body contours L0 L1 A0 L2 A1 L3 A2 L4 A3 L5 L18 L19 L20 A23 L21 A24 L22 A25 L23 A26 L24 L25 makes body 3
extrude "Extrusion12" add sketch "Skizze4" against normal blind 2.4 contours L6 L7 A4 L8 A5 L9 A6 L10 A7 L12 L18 L19 L20 A23 L21 A24 L22 A25 L23 A26 L24 L25 bodies 3
extrude "Extrusion13" add sketch "Skizze4" against normal blind 7.7 separate body contours A9 | A10 | A20 | A22 makes body 4 at (-1.5037, 7.3505, 4.4667) makes body 5 at (37.4963, 7.3505, 4.4667)
extrude "Extrusion14" add sketch "Skizze4" against normal blind 6.1 separate body contours A8 | A18 makes body 6
combine "Kombinieren1" operation add target body 2 tool bodies 3 4 5 6
extrude "Extrusion15" add sketch "Skizze4" against normal blind 3.4 contours L0 L18 L19 L25 | L6 L18 L19 L25 bodies 2
equation "d5 = d4"
equation "d36 = d35"
equation "d37 = d34"
named bodies: "bottom shell CP", "top shell CP"
